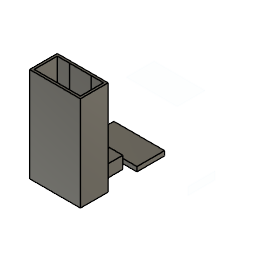
modelo_v3 (Autodesk Fusion 360 archive; units mm, degrees)
design "Contorno"
part number: 2026-06-03-17-36-54-993
Autodesk Fusion 360 part; units mm, degrees
note: some values were not read from the file. Chosen so that the rebuilt part matches the saved one: which bodies a step acts on.
sketch "Boceto1" plane through (0, 0, 0) normal (0, 0, 1) x (1, 0, 0)
  line L0 (0, 0) -> (60, 0)
  line L1 (60, 0) -> (60, 30)
  line L2 (0, 30) -> (0, 0)
  line L3 (44, 30) -> (44, 65)
  line L4 (44, 65) -> (16, 65)
  line L5 (16, 65) -> (16, 30)
  line L6 (0, 30) -> (16, 30)
  line L7 (44, 30) -> (60, 30)
  line L8 (13, 68) -> (13, 33)
  line L9 (-3, 33) -> (13, 33)
  line L10 (-3, 33) -> (-3, -3)
  line L11 (-3, -3) -> (63, -3)
  line L12 (63, -3) -> (63, 33)
  line L13 (47, 33) -> (63, 33)
  line L14 (47, 33) -> (47, 68)
  line L15 (47, 68) -> (13, 68)
  dimension "d1" = 60
  dimension "d2" = 30
  dimension "d3" = 35
  dimension "d4" = 28
  dimension "d5" = 16
  dimension "d6" = 16
  dimension "d7" = -3
  constraint horizontal L0
  constraint vertical L1
  constraint vertical L2
  constraint coincident L0.start L2.end
  constraint vertical L3
  constraint horizontal L4
  constraint vertical L5
  measures "d1" distance of L0.start L0.end
  measures "d2" distance of L0.start L2.start
  measures "d3" distance of L5.end L4.end
  measures "d4" distance of L3.end L4.end
  measures "d5" distance of L1.end L3.start
  measures "d6" distance of L2.start L5.end
extrude "Extruir1" add sketch "Boceto1" along normal blind 3 contours L0 L1 L2 L3 L4 L5 L6 L7 | L8 L9 L10 L11 L12 L13 L14 L15 makes body 1
sketch "Boceto2" plane through (0, 0, 0) normal (0, 0, -1) x (1, 0, 0)
  line L0 (47, -68) -> (47, -33)
  line L1 (47, -33) -> (63, -33)
  line L2 (63, -33) -> (63, 3)
  line L3 (63, 3) -> (-3, 3)
  line L4 (-3, 3) -> (-3, -33)
  line L5 (-3, -33) -> (13, -33)
  line L6 (13, -33) -> (13, -68)
  line L7 (13, -68) -> (47, -68)
  line L8 (16, -30) -> (16, -65)
  line L9 (16, -65) -> (44, -65)
  line L10 (44, -65) -> (44, -30)
  line L11 (44, -30) -> (60, -30)
  line L12 (60, -30) -> (60, 0)
  line L13 (60, 0) -> (0, 0)
  line L14 (0, 0) -> (0, -30)
  line L15 (0, -30) -> (16, -30)
  dimension "d10" = -3
extrude "Extruir2" add sketch "Boceto2" along normal blind 10 bodies 1
sketch "Boceto4" plane through (0, 0, 3) normal (0, 0, 1) x (-1, 0, 0)
  line L0 (-47, -33) -> (-47, -68)
  line L1 (-47, -68) -> (-13, -68)
  line L2 (-13, -68) -> (-13, -33)
  line L3 (-13, -33) -> (3, -33)
  line L4 (3, -33) -> (3, 3)
  line L5 (3, 3) -> (-63, 3)
  line L6 (-63, 3) -> (-63, -33)
  line L7 (-63, -33) -> (-47, -33)
  line L8 (-13, -33) -> (-47, -33)
  constraint coincident L2.end L3.start
  constraint coincident L0.start L7.end
extrude "Extruir3" add sketch "Boceto4" along normal blind 113 contours L3 L4 L5 L6 L7 L8 bodies 1
sketch "Boceto5" plane through (0, 0, 116) normal (0, 0, 1) x (-1, 0, 0)
  line L0 (3, -33) -> (3, 3)
  line L1 (3, 3) -> (-63, 3)
  line L2 (-63, 3) -> (-63, -33)
  line L3 (-63, -33) -> (-47, -33)
  line L4 (-47, -33) -> (-13, -33)
  line L5 (-13, -33) -> (3, -33)
sketch "Boceto3" plane through (0, 0, 0) normal (0, 0, -1) x (1, 0, 0)
  line L0 (16, -30) -> (16, -65)
  line L1 (16, -65) -> (44, -65)
  line L2 (44, -65) -> (44, -30)
  line L3 (44, -30) -> (60, -30)
  line L4 (60, -30) -> (60, 0)
  line L5 (60, 0) -> (0, 0)
  line L6 (0, 0) -> (0, -30)
  line L7 (0, -30) -> (16, -30)
  line L8 (44, -30) -> (16, -30)
  line L9 (44, -30) -> (60, -30)
  line L10 (60, -30) -> (60, 0)
  line L11 (60, 0) -> (0, 0)
  line L12 (16, -30) -> (0, -30)
  line L13 (0, -30) -> (0, 0)
  line L14 (0, -30) -> (0, 0)
  line L15 (0, 0) -> (60, 0)
  line L16 (60, 0) -> (60, -30)
  constraint coincident L2.end L3.start
  constraint coincident L0.start L7.end
  constraint coincident L3.end L4.start
  constraint coincident L4.end L5.start
  constraint coincident L5.end L6.start
  constraint coincident L6.end L7.start
  constraint vertical L14
  constraint horizontal L15
  constraint vertical L16
extrude "Extruir4" cut sketch "Boceto3" against normal blind 110 contours L3 L4 L5 L6 L7 L8 L9 L10 L11 L12 L13 L14 L15 L16 bodies 1
extrude "Extruir5" add 1 faces at (20, -2, -10) along direction (0, 0, -1) blind 5 on bodies 1 bodies 1
sketch "Boceto6" plane through (0, 0, -15) normal (0, 0, -1) x (1, 0, 0)
  line L0 (16, -30) -> (0, -30)
  line L1 (0, -30) -> (0, 0)
  line L2 (0, 0) -> (60, 0)
  line L3 (60, 0) -> (60, -30)
  line L4 (60, -30) -> (44, -30)
  line L5 (44, -30) -> (44, -65)
  line L6 (44, -65) -> (16, -65)
  line L7 (16, -65) -> (16, -30)
  line L8 (13, -68) -> (47, -68)
  line L9 (47, -68) -> (47, -33)
  line L10 (47, -33) -> (63, -33)
  line L11 (63, -33) -> (63, 3)
  line L12 (63, 3) -> (-3, 3)
  line L13 (-3, 3) -> (-3, -33)
  line L14 (-3, -33) -> (13, -33)
  line L15 (13, -33) -> (13, -68)
  line L16 (14.5, -66.5) -> (14.5, -31.5)
  line L17 (14.5, -31.5) -> (-1.5, -31.5)
  line L18 (-1.5, -31.5) -> (-1.5, 1.5)
  line L19 (-1.5, 1.5) -> (61.5, 1.5)
  line L20 (61.5, 1.5) -> (61.5, -31.5)
  line L21 (61.5, -31.5) -> (45.5, -31.5)
  line L22 (45.5, -31.5) -> (45.5, -66.5)
  line L23 (45.5, -66.5) -> (14.5, -66.5)
  dimension "d19" = -1.5
extrude "Extruir6" cut sketch "Boceto6" against normal blind 5 contours L16 L17 L18 L19 L20 L21 L22 L23 bodies 1
extrude "Extruir7" cut 1 faces at (19.5, -2.5, -15) along direction (0, 0, 1) blind 2 on bodies 1 bodies 1
sketch "Boceto7" plane through (0, 0, 0) normal (0, 0, -1) x (1, 0, 0)
  line L0 (44, -30) -> (16, -30)
  line L1 (16, -30) -> (16, -65)
  line L2 (16, -65) -> (44, -65)
  line L3 (44, -65) -> (44, -30)
  line L4 (44, -31) -> (16, -31)
  dimension "d24" = -1
extrude "Extruir8" add sketch "Boceto7" along normal blind 1 contours L0 L1 L3 L4 bodies 1
sketch "Boceto8" plane through (44, 0, 0) normal (-1, 0, 0) x (0, -1, 0)
  line L0 (-31, -1) -> (-31, 0)
  line L1 (-31, 0) -> (-65, 0)
  line L2 (-65, 0) -> (-65, -10)
  line L3 (-65, -10) -> (-30, -10)
  line L4 (-30, -10) -> (-30, -1)
  line L5 (-30, -1) -> (-31, -1)
extrude "Extruir9" cut 1 faces at (34.6667, 31, -0.3333) along direction (0, -1, 0) blind 0.5 on bodies 1 bodies 1
sketch "Boceto9" plane through (44, 0, 0) normal (-1, 0, 0) x (0, -1, 0)
  line L0 (-30.5, -1) -> (-30.5, -10)
  line L1 (-30.5, -1) -> (-30, -1)
  line L2 (-30, -1) -> (-30, -10)
  line L3 (-30, -10) -> (-30.5, -10)
  line L4 (-30.5, -10) -> (-30.5, -1)
  constraint vertical L0
  constraint horizontal L1
  constraint vertical L2
  constraint horizontal L3
  constraint vertical L4
extrude "Extruir10" add sketch "Boceto9" along normal blind 0.5 bodies 1
sketch "Boceto10" plane through (16, 0, 0) normal (1, 0, 0) x (0, 1, 0)
  line L0 (31, 0) -> (31, -1)
  line L1 (31, -1) -> (30.5, -1)
  line L2 (30.5, -1) -> (30, -1)
  line L3 (30, -1) -> (30, -10)
  line L4 (30, -10) -> (65, -10)
  line L5 (65, -10) -> (65, 0)
  line L6 (65, 0) -> (31, 0)
  line L7 (30.5, -1) -> (30, -1)
  line L8 (30, -1) -> (30, -10)
  line L9 (30, -10) -> (30.5, -10)
  line L10 (30.5, -10) -> (30.5, -1)
  constraint horizontal L7
  constraint vertical L8
  constraint horizontal L9
  constraint vertical L10
  constraint coincident L3.end L4.start
  constraint coincident L1.end L2.start
extrude "Extruir11" add sketch "Boceto10" along normal blind 0.5 contours L2 L3 L4 L7 L8 L9 L10 bodies 1
sketch "Boceto11" plane through (0, 0, 0) normal (0, 0, -1) x (1, 0, 0)
  line L0 (16, -31) -> (16, -65)
  line L1 (16, -65) -> (44, -65)
  line L2 (44, -65) -> (44, -31)
  line L3 (44, -31) -> (44, -30.5)
  line L4 (44, -30.5) -> (16, -30.5)
  line L5 (16, -30.5) -> (16, -31)
  line L6 (44, -31.5) -> (16, -31.5)
  line L7 (44, -31.5) -> (16, -31.5)
  line L8 (16, -31.5) -> (16, -32)
  line L9 (16, -32) -> (44, -32)
  line L10 (44, -32) -> (44, -31.5)
  dimension "d33" = -1
  dimension "d34" = 0.5
  constraint horizontal L7
  constraint vertical L8
  constraint horizontal L9
  constraint vertical L10
  constraint coincident L0 L8.end
  measures "d34" distance of L6.start L9.end
extrude "Extruir12" add sketch "Boceto11" along normal blind 0.5 contours L0 L2 L6 L7 L8 L9 L10 bodies 1
sketch "Boceto12" plane through (44, 0, 0) normal (-1, 0, 0) x (0, -1, 0)
  line L0 (-31.5, -0.5) -> (-32, -0.5)
  line L1 (-32, -0.5) -> (-32, -10)
  line L2 (-32, -10) -> (-31.5, -10)
  line L3 (-31.5, -10) -> (-31.5, -0.5)
  constraint horizontal L0
  constraint vertical L1
  constraint horizontal L2
  constraint vertical L3
extrude "Extruir13" add sketch "Boceto12" along normal blind 0.5 bodies 1
sketch "Boceto13" plane through (16, 0, 0) normal (1, 0, 0) x (0, 1, 0)
  line L0 (32, 0) -> (32, -0.5)
  line L1 (32, -0.5) -> (31.5, -0.5)
  line L2 (31.5, -0.5) -> (31.5, 0)
  line L3 (31.5, 0) -> (31, 0)
  line L4 (31, 0) -> (31, -1)
  line L5 (31, -1) -> (30.5, -1)
  line L6 (30.5, -1) -> (30.5, -10)
  line L7 (30.5, -10) -> (65, -10)
  line L8 (65, -10) -> (65, 0)
  line L9 (65, 0) -> (32, 0)
  line L10 (32, -0.5) -> (31.5, -0.5)
  line L11 (31.5, -0.5) -> (31.5, -10)
  line L12 (31.5, -10) -> (32, -10)
  line L13 (32, -10) -> (32, -0.5)
  constraint horizontal L10
  constraint vertical L11
  constraint horizontal L12
  constraint vertical L13
  constraint coincident L7 L11.end
  constraint coincident L0.end L1.start
extrude "Extruir14" add sketch "Boceto13" along normal blind 0.5 contours L1 L7 L10 L11 L12 L13 bodies 1
move_body "Desplazar1" bodies 1 to x (1, 0, 0) y (0, 1, 0) z (0, 0, 1) at (-70, -60, 10)
split "Dividir1" by plane through (-70, -60, 120) normal (0, 0, -1) bodies 1 makes body 2 at (-29, -63, 79)
move_body "Desplazar2" bodies 1 to x (1, 0, 0) y (0, 1, 0) z (0, 0, 1) at (0, 50, 0)
move_body "Desplazar3" bodies 1 to x (1, 0, 0) y (0, 1, 0) z (0, 0, 1) at (0, 0, -80)
move_body "Desplazar4" bodies 1 to x (1, 0, 0) y (0, 1, 0) z (0, 0, 1) at (0, 40, -10)
move_body "Desplazar5" bodies 1 to x (1, 0, 0) y (0, 1, 0) z (0, 0, 1) at (73, -63, -30)
move_body "Desplazar6" bodies 2 to x (1, 0, 0) y (0, 1, 0) z (0, 0, 1) at (89, -44, 3)
move_body "Desplazar7" bodies 2 to x (1, 0, 0) y (0, 1, 0) z (0, 0, 1) at (0, -10, 0)
move_body "Desplazar8" bodies 1 to x (1, 0, 0) y (0, 1, 0) z (0, 0, 1) at (-71.6342, 49.3695, 0)
move_body "Desplazar9" bodies 2 to x (1, 0, 0) y (0, 1, 0) z (0, 0, 1) at (-83.5732, 52.919, 0)
